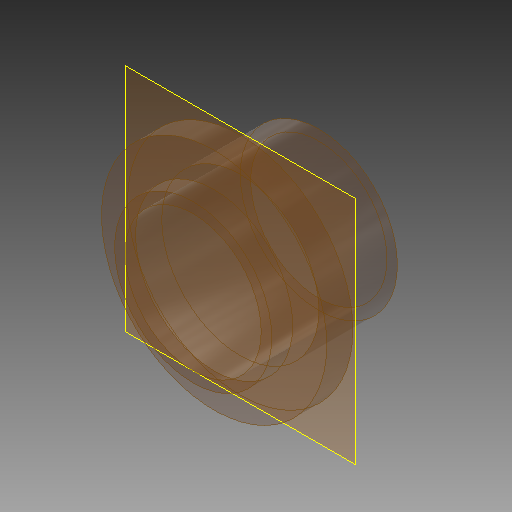
# Autodesk Inventor part: Adaptador de Saida
Saved by Autodesk Inventor 2019 (Build 230136000, 136)
## iProperties
Created: 2020-04-02
Part Number: Adaptador de Saida
Material: Genérico
Document SubType Name: Modeling
Designer: Paulo Rodrigues
Density: 1 g/cm^3
Appearance: Policarbonato - Fumê
Author: Paulo Rodrigues
Autodesk Inventor part; units mm, degrees
ref_plane "YZ Plane" through (0, 0, 0) normal (1, 0, 0) x (0, 1, 0)
ref_plane "XZ Plane" through (0, 0, 0) normal (0, 1, 0) x (-1, 0, 0)
ref_plane "XY Plane" through (0, 0, 0) normal (0, 0, 1) x (1, 0, 0)
ref_plane "Plano de trabalho1" through (0, 0, 0) normal (0, 0, 1) x (1, 0, 0)
sketch "Esboço1" plane through (0, 0, 0) normal (0, 0, 1) x (1, 0, 0)
  circle A0 centre (-15, 0) radius 15 projected
  circle A1 centre (-15, 0) radius 13
  point P0 (0, 0)
  dimension "d0" = 2
  constraints: 1 centre point, 1 horizontal alignment
extrude "Extrusão1" add sketch "Esboço1" against normal blind 15
sketch "Esboço2" plane through (-15, 0, 0) normal (0, 0, 1) x (1, 0, 0)
  circle A0 centre (0, 0) radius 13 projected
  circle A1 centre (0, 0) radius 20 projected
  circle A2 centre (0, 0) radius 21.5
  point P0 (15, 0)
  dimension "d3" = 43
  constraints: 1 centre point, 1 coincident
  measures "d3" diameter of A2
extrude "Extrusão2" add sketch "Esboço2" along normal blind 5 contours A1 | A2
sketch "Esboço3" plane through (-15, 0, 5) normal (0, 0, 1) x (1, 0, 0)
  circle A0 centre (0, 0) radius 13 projected
  circle A1 centre (0, 0) radius 15 projected
  point P0 (15, 0)
  constraints: 1 horizontal alignment
extrude "Extrusão3" add sketch "Esboço3" along normal blind 4
